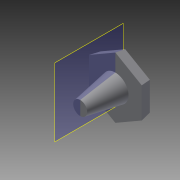
# Autodesk Inventor part: Driver Shaft Cap
Saved by Autodesk Inventor 2018 (Build 220112000, 112)
## iProperties
Created: 2018-01-21
Part Number: Driver Shaft Cap
Material: Generic
Document SubType Name: Modeling
Designer: Rus
Density: 1 g/cm^3
Appearance: Default
Author: Rus
Autodesk Inventor part; units mm, degrees
ref_plane "YZ Plane" through (0, 0, 0) normal (1, 0, 0) x (0, 1, 0)
ref_plane "XZ Plane" through (0, 0, 0) normal (0, 1, 0) x (-1, 0, 0)
ref_plane "XY Plane" through (0, 0, 0) normal (0, 0, 1) x (1, 0, 0)
sketch "Sketch1" plane through (0, 0, 0) normal (0, 0, 1) x (1, 0, 0)
  line L0 (5.644444, -5.644444) -> (-5.644444, -5.644444)
  line L1 (-5.644444, -5.644444) -> (-5.644444, 5.644444)
  line L2 (-5.644444, 5.644444) -> (5.644444, 5.644444)
  line L3 (5.644444, 5.644444) -> (5.644444, -5.644444)
  point P0 (0, 0)
  point P1 (0, 0)
  dimension "d0" = 11.28889
  constraints: 8 end point, 1 coincident, 1 horizontal, 9 other
  measures "d0" distance of L1.end L2.end
extrude "Extrusion1" add sketch "Sketch1" along normal blind 8.466667
ref_plane "Work Plane1" through (0, 5.644444, 8.466667) normal (-1, 0, 0) x (0, -1, 0)
sketch "Sketch2" plane through (0, 5.644444, 8.466667) normal (-1, 0, 0) x (0, -1, 0)
  line L0 (5.644444, -8.466667) -> (-2.822222, -8.466667)
  line L1 (0, -8.466667) -> (11.288889, -8.466667)
  line L2 (5.644444, -8.466667) -> (5.644444, -11.641667)
  arc A0 (-2.822222, -8.466667) -> (5.644444, -11.641667) centre (5.644444, 1.234722) ccw
  dimension "d3" = 8.46667
  dimension "d4" = 3.175
  constraints: 4 end point, 2 point on circle, 1 centre point, 1 collinear, 1 line through centre, 1 vertical
  measures "d3" distance of L0.start L0.end
  measures "d4" distance of L0.start L2.end
revolve "Revolution1" add sketch "Sketch2" angle 360 about axis through (0, 0, 0) along (0, 0, -1)
sketch "Sketch3" plane through (0, 0, 8.466667) normal (0, 0, 1) x (1, 0, 0)
  line L0 (-5.644444, -5.644444) -> (5.644444, -5.644444)
  line L1 (5.644444, -5.644444) -> (5.644444, 5.644444)
  line L2 (5.644444, 5.644444) -> (-5.644444, 5.644444)
  line L3 (-5.644444, 5.644444) -> (-5.644444, -5.644444)
  point P0 (0, 0)
extrude "Extrusion2" cut sketch "Sketch3" against normal up to surface (8.466667 mm away)
sketch "Sketch4" plane through (0, 0, 0) normal (0, 0, 1) x (1, 0, 0)
  circle A0 centre (0, 0) radius 4.233333
  dimension "d8" = 8.46667
  constraints: 1 centre point, 1 coincident
  measures "d8" diameter of A0
extrude "Extrusion3" add sketch "Sketch4" along normal blind 11.288889 draft -10
sketch "Sketch5" plane through (0, 0, 0) normal (0, 0, 1) x (1, 0, 0)
  circle A0 centre (0, 0) radius 8.466667
  line L0 (8.466667, -4.888232) -> (0, -9.776465)
  line L1 (0, -9.776465) -> (-8.466667, -4.888232)
  line L2 (-8.466667, -4.888232) -> (-8.466667, 4.888232)
  line L3 (-8.466667, 4.888232) -> (0, 9.776465)
  line L4 (0, 9.776465) -> (8.466667, 4.888232)
  line L5 (8.466667, 4.888232) -> (8.466667, -4.888232)
  point P0 (0, 0)
  point P1 (0, 0)
  point P2 (8.466667, 0)
  constraints: 12 end point, 1 coincident, 1 horizontal alignment, 1 midpoint, 1 vertical, 14 other
sketch "Sketch5 outline for Extrusion4" plane through (0, 0, 0) normal (0, 0, 1) x (1, 0, 0)
  line L0 (8.466667, 0) -> (8.466667, -4.888232)
  line L1 (8.466667, -4.888232) -> (0, -9.776465)
  line L2 (0, -9.776465) -> (-8.466667, -4.888232)
  line L3 (-8.466667, -4.888232) -> (-8.466667, 4.888232)
  line L4 (-8.466667, 4.888232) -> (0, 9.776465)
  line L5 (0, 9.776465) -> (8.466667, 4.888232)
  line L6 (8.466667, 4.888232) -> (8.466667, 0)
extrude "Extrusion4" add sketch "Sketch5 outline for Extrusion4" against normal blind 3.175 draft -10
body "Solid1"
